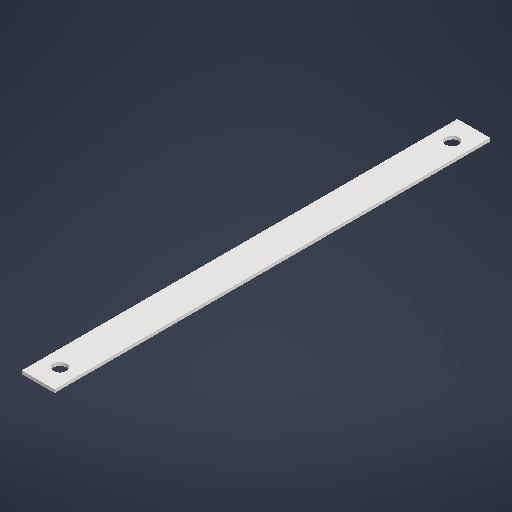
# Autodesk Inventor part: rig_connector_long
Saved by Autodesk Inventor 2027.1 (Build 311270010, 270A)
## iProperties
Created: 2026-09-04
Part Number: rig_connector_long
Material: Generic
Document SubType Name: Modeling
Designer: ajrcr
Density: 1 g/cm^3
Appearance: Default
Author: ajrcr
Autodesk Inventor part; units mm, degrees
ref_plane "YZ Plane" through (0, 0, 0) normal (1, 0, 0) x (0, 1, 0)
ref_plane "XZ Plane" through (0, 0, 0) normal (0, 1, 0) x (-1, 0, 0)
ref_plane "XY Plane" through (0, 0, 0) normal (0, 0, 1) x (1, 0, 0)
sketch "Sketch1" plane through (0, 0, 0) normal (0, 1, 0) x (-1, 0, 0)
  line L0 (65, 90) -> (35, 90)
  line L1 (35, 90) -> (35, -310)
  line L2 (35, -310) -> (65, -310)
  line L3 (65, -310) -> (65, 90)
  line L4 (50, 90) -> (50, -310) construction
  circle A0 centre (50, 70) radius 6
  circle A1 centre (50, -290) radius 6
  point P0 (0, 0)
  dimension "d0" = 30
  dimension "d1" = 400
  dimension "d2" = 35
  dimension "d3" = 90
  dimension "d6" = 12
  dimension "d7" = 12
  dimension "d8" = 20
  dimension "d9" = 20
  constraints: 10 end point, 2 centre point, 2 midpoint, 2 parallel, 2 point on line, 1 horizontal, 1 perpendicular
  measures "d0" distance of L2.end L1.end
  measures "d1" distance of L1.end L0.end
  measures "d2" distance from line of point (0, 0) L1
  measures "d3" vertical distance of point (0, 0) L4.start
  measures "d6" diameter of A0
  measures "d7" diameter of A1
  measures "d8" distance from line of L0 A0.centre
  measures "d9" distance from line of L2 A1.centre
extrude "Extrusion1" add sketch "Sketch1" along normal blind 3
body "Solid1"
